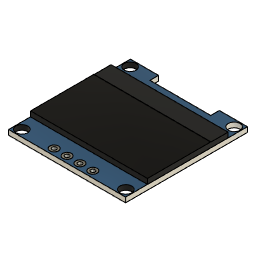
Ticker Tracker 2.0 (Autodesk Fusion 360 archive; units mm, degrees)
design "I2C OLED"
Autodesk Fusion 360 part; units mm, degrees
sketch "Sketch1" plane through (0, 0, 0) normal (0, 0, 1) x (1, 0, 0)
  line L0 (13.6, 14.175) -> (-13.6, 14.175)
  line L1 (-13.6, 14.175) -> (-13.6, -14.175)
  line L2 (-13.6, -14.175) -> (13.6, -14.175)
  line L3 (13.6, -14.175) -> (13.6, 14.175)
  line L4 (13.6, 14.175) -> (-13.6, -14.175) construction
  line L5 (-13.6, 14.175) -> (13.6, -14.175) construction
  line L6 (-7.075, 14.175) -> (7.075, 14.175)
  line L7 (7.075, 14.175) -> (7.075, 12.175)
  line L8 (7.075, 12.175) -> (-7.075, 12.175)
  line L9 (-7.075, 12.175) -> (-7.075, 14.175)
  line L10 (-13.6, 9.675) -> (13.6, 9.675)
  line L11 (13.6, 9.675) -> (13.6, -9.075)
  line L12 (13.6, -9.075) -> (-13.6, -9.075)
  line L13 (-13.6, -9.075) -> (-13.6, 9.675)
  line L14 (-13.6, 5.675) -> (13.6, 5.675)
  circle A0 centre (12.0919, 12.6032) radius 1.375
  circle A1 centre (-4.5, -12.675) radius 1
  circle A2 centre (-4.5, -12.675) radius 1
  circle A3 centre (-1.5, -12.675) radius 1
  circle A4 centre (1.5, -12.675) radius 1
  circle A5 centre (4.5, -12.675) radius 1
  line L15 (-4.5, -12.675) -> (4.5, -12.675) construction
  line L16 (0, -14.175) -> (0, -11.175) construction
  circle A6 centre (-4.5, -12.675) radius 0.5
  circle A7 centre (-1.5, -12.675) radius 0.5
  circle A8 centre (1.5, -12.675) radius 0.5
  circle A9 centre (4.5, -12.675) radius 0.5
  circle A10 centre (-12.1081, 12.6032) radius 1.375
  circle A11 centre (12.0919, -12.5968) radius 1.375
  circle A12 centre (-12.1081, -12.5968) radius 1.375
  dimension "d1" = 27.2
  dimension "d2" = 28.35
  dimension "d3" = 14.15
  dimension "d4" = 2
  dimension "d5" = 18.75
  dimension "d6" = 4.5
  dimension "d7" = 4
  dimension "d8" = 2.75
  dimension "d22" = 2
  dimension "d23" = 2
  dimension "d26" = 3
  dimension "d27" = 0
  dimension "d30" = 3
  dimension "d31" = 1
  dimension "d36" = -24.2
  dimension "d37" = -25.2
  constraint horizontal L0
  constraint perpendicular L0 L1
  constraint parallel L0 L2
  constraint parallel L1 L3
  constraint coincident L4 origin
  constraint coincident L5 origin
  constraint horizontal L6
  constraint vertical L7
  constraint horizontal L8
  constraint vertical L9
  constraint midpoint L0 L6
  constraint horizontal L10
  constraint vertical L11
  constraint horizontal L12
  constraint vertical L13
  constraint coincident L1 L10.start
  constraint coincident L3 L10.end
  constraint coincident L13 L14.start
  constraint coincident L3 L14.end
  constraint perpendicular L3 L14
  constraint coincident A1.centre A2.centre
  constraint coincident A5.centre L15.end
  constraint horizontal L15
  constraint midpoint L2 L16.start
  constraint perpendicular L15 L16
  constraint midpoint L15 L16
  constraint concentric A2 A6
  constraint coincident L4 A0.centre
  measures "d1" distance of L1.end L2.end
  measures "d2" distance of L0.end L1.end
  measures "d3" distance of L6.start L6.end
  measures "d4" distance of L6.start L8.end
  measures "d5" distance of L10.start L12.end
  measures "d6" distance of L0 L10
  measures "d7" distance of L10 L14
  measures "d8" diameter of A0
  measures "d22" diameter of A1
  measures "d23" diameter of A2
  measures "d30" distance of L16.start L16.end
  measures "d31" diameter of A6
extrude "Extrude1" add sketch "Sketch1" against normal blind 1.15 contours L0 L1 L3 L7 L8 L9 L10 | L1 L3 L10 L11 L13 L14 | L1 L3 L11 L12 L13 L14 | L1 L2 L3 L12 | A1 A2 | A3 | A4 | A5
extrude "Extrude2" add sketch "Sketch1" along normal blind 1.15 contours L1 L3 L10 L11 L13 L14
extrude "Extrude3" add sketch "Sketch1" along normal blind 1.2 contours L1 L3 L11 L12 L13 L14
sketch "Sketch2" plane through (13.6, 0, 0) normal (1, 0, 0) x (0, 1, 0)
  line L0 (-9.075, 0) -> (-14.175, 0)
  line L1 (-14.175, 0) -> (-14.175, -1.15)
  line L2 (-14.175, -1.15) -> (14.175, -1.15)
  line L3 (14.175, -1.15) -> (14.175, 0)
  line L4 (14.175, 0) -> (9.675, 0)
  line L5 (9.675, 0) -> (9.675, 1.15)
  line L6 (9.675, 1.15) -> (5.675, 1.15)
  line L7 (5.675, 1.15) -> (5.675, 1.2)
  line L8 (5.675, 1.2) -> (-9.075, 1.2)
  line L9 (-9.075, 1.2) -> (-9.075, 0)
  line L10 (-9.075, 0) -> (9.675, 0)
  constraint coincident L0.start L9.end
  constraint coincident L4.end L5.start
extrude "Extrude4" add sketch "Sketch2" along normal blind 0.01 contours L0 L1 L2 L3 L4 L10
sketch "Sketch3" plane through (-13.6, 0, 0) normal (-1, 0, 0) x (0, -1, 0)
  line L0 (-9.675, 0) -> (-14.175, 0)
  line L1 (-14.175, 0) -> (-14.175, -1.15)
  line L2 (-14.175, -1.15) -> (14.175, -1.15)
  line L3 (14.175, -1.15) -> (14.175, 0)
  line L4 (14.175, 0) -> (9.075, 0)
  line L5 (9.075, 0) -> (9.075, 1.2)
  line L6 (9.075, 1.2) -> (-5.675, 1.2)
  line L7 (-5.675, 1.2) -> (-5.675, 1.15)
  line L8 (-5.675, 1.15) -> (-9.675, 1.15)
  line L9 (-9.675, 1.15) -> (-9.675, 0)
  line L10 (-9.675, 0) -> (9.075, 0)
  constraint coincident L0.start L9.end
  constraint coincident L4.end L5.start
extrude "Extrude5" add sketch "Sketch3" along normal blind 0.01 contours L0 L1 L2 L3 L4 L10
extrude "Extrude6" cut sketch "Sketch1" against normal blind 0.01 contours A1 A2 | A3 | A4 | A5
equation "d26 = 1 mm + 2 mm"
